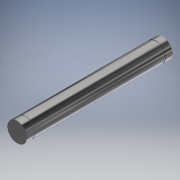
# Autodesk Inventor part: Mecanum Axle
Saved by Autodesk Inventor 2019.4 (Build 234330000, 330)
## iProperties
Created: 2019-11-02
Part Number: Mecanum Axle
Material: Stainless Steel
Document SubType Name: Modeling
Designer: admin
Density: 8 g/cm^3
Appearance: Semi-Polished
Author: admin
Autodesk Inventor part; units mm, degrees
ref_plane "YZ Plane" through (0, 0, 0) normal (1, 0, 0) x (0, 1, 0)
ref_plane "XZ Plane" through (0, 0, 0) normal (0, 1, 0) x (-1, 0, 0)
ref_plane "XY Plane" through (0, 0, 0) normal (0, 0, 1) x (1, 0, 0)
sketch "Sketch1" plane through (0, 0, 0) normal (1, 0, 0) x (0, 1, 0)
  line L0 (7.5, 0) -> (7.5, -5.3)
  line L1 (7.5, -5.3) -> (7.15, -5.3)
  line L2 (7.15, -5.3) -> (7.15, -6.4)
  line L3 (7.15, -6.4) -> (7.5, -6.4)
  line L4 (7.5, -6.4) -> (7.5, -105.8)
  line L5 (7.5, -105.8) -> (7.15, -105.8)
  line L6 (7.15, -105.8) -> (7.15, -106.9)
  line L7 (7.15, -106.9) -> (7.5, -106.9)
  line L8 (7.5, -106.9) -> (7.5, -112.2)
  line L9 (7.5, -112.2) -> (0, -112.2)
  line L10 (0, -112.2) -> (0, 0)
  line L11 (0, 0) -> (7.5, 0)
  dimension "d0" = 0.35
  dimension "d1" = 1.1
  dimension "d2" = 7.5
  dimension "d3" = 5.3
  dimension "d4" = 5.3
  dimension "d5" = 1.1
  dimension "d6" = 112.2
  constraints: 24 end point, 8 perpendicular, 6 point on line, 1 coincident, 1 vertical
  measures "d0" distance of L0.end L1.end
  measures "d1" distance of L1.end L2.end
  measures "d2" distance of L10.end L0.start
  measures "d3" distance of L0.start L0.end
  measures "d4" distance of L7.end L8.end
  measures "d5" distance of L5.end L6.end
  measures "d6" distance of L9.end L10.end
revolve "Revolution1" add sketch "Sketch1" angle 360 about axis through (0, 0, -112.2) along (0, 0, 1)
sketch "Sketch2" plane through (0, 0, 0) normal (0, 1, 0) x (-1, 0, 0)
  circle A0 centre (0, -74.4) radius 3.25
  line L0 (0, -74.4) -> (0, -112.2) construction
  line L1 (-7.5, -112.2) -> (7.5, -112.2) projected
  point P0 (0, 0)
  dimension "d8" = 6.5
  dimension "d9" = 37.8
  constraints: 2 end point, 1 centre point, 1 midpoint, 1 vertical
  measures "d8" diameter of A0
  measures "d9" distance of L0.start L0.end
extrude "Extrusion1" cut sketch "Sketch2" against normal blind 10
sketch "Sketch3" plane through (0, 0, -74.4) normal (0, -1, 0) x (1, 0, 0)
  circle A0 centre (0, -22.2) radius 3.25
  line L0 (-7.5, -37.8) -> (7.5, -37.8) projected
  line L1 (0, -22.2) -> (0, -37.8) construction
  point P0 (0, 74.4)
  dimension "d12" = 6.5
  dimension "d13" = 15.6
  constraints: 2 end point, 1 centre point, 1 midpoint, 1 vertical
  measures "d12" diameter of A0
  measures "d13" distance from line of L0 L1.start
extrude "Extrusion2" cut sketch "Sketch3" along normal blind 10
body "Solid1"
